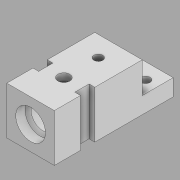
# Autodesk Inventor part: Box A01209499
Saved by Autodesk Inventor 2020 (Build 240168000, 168)
## iProperties
Created: 2019-10-15
Part Number: Box A01209499
Material: Genérico
Document SubType Name: Modeling
Designer: gerar
Density: 1 g/cm^3
Appearance: Valor por defecto
Author: gerar
Autodesk Inventor part; units mm, degrees
ref_plane "YZ Plane" through (0, 0, 0) normal (1, 0, 0) x (0, 1, 0)
ref_plane "XZ Plane" through (0, 0, 0) normal (0, 1, 0) x (-1, 0, 0)
ref_plane "XY Plane" through (0, 0, 0) normal (0, 0, 1) x (1, 0, 0)
sketch "Boceto1" plane through (0, 0, 0) normal (0, 1, 0) x (-1, 0, 0)
  line L0 (0, 0) -> (50.8, 0)
  line L1 (50.8, -93.98) -> (0, -93.98)
  line L2 (50.8, -27.94) -> (44.704, -27.94)
  line L3 (44.704, -27.94) -> (44.704, -43.18)
  line L4 (44.704, -43.18) -> (50.8, -43.18)
  line L5 (6.096, -27.94) -> (0, -27.94)
  line L6 (0, -43.18) -> (6.096, -43.18)
  line L7 (6.096, -43.18) -> (6.096, -27.94)
  line L8 (50.8, 0) -> (50.8, -27.94)
  line L9 (50.8, -43.18) -> (50.8, -93.98)
  line L10 (0, -93.98) -> (0, -43.18)
  line L11 (0, -27.94) -> (0, 0)
  dimension "d0" = 50.8
  dimension "d1" = 93.98
  dimension "d2" = 27.94
  dimension "d3" = 15.24
  dimension "d5" = 27.94
  dimension "d6" = 15.24
  constraints: 24 end point, 7 parallel, 3 horizontal, 3 perpendicular, 1 point on line
  measures "d0" distance of L1.start L1.end
  measures "d1" distance of L0.end L1.start
  measures "d2" distance between parallel lines of L0 L2
  measures "d3" distance between parallel lines of L2 L4
  measures "d5" distance between parallel lines of L0 L5
  measures "d6" distance between parallel lines of L6 L5
extrude "BaseAlta" add sketch "Boceto1" along normal blind 50.8
sketch "Boceto2" plane through (0, 0, 0) normal (0, 1, 0) x (-1, 0, 0)
  line L0 (0, -93.98) -> (50.8, -93.98) projected
  line L1 (0, -93.98) -> (50.8, -93.98)
  line L2 (50.8, -93.98) -> (50.8, -127)
  line L3 (50.8, -127) -> (0, -127)
  line L4 (0, -127) -> (0, -93.98)
  point P0 (0, 0)
  dimension "d10" = 50.8
  dimension "d11" = 33.02
  constraints: 8 end point, 2 parallel, 1 horizontal, 1 perpendicular
  measures "d10" distance of L2.end L3.end
  measures "d11" distance of L1.end L2.end
extrude "BaseBaja" add sketch "Boceto2" along normal blind 17.78
sketch "Boceto4" plane through (0, 50.8, -93.98) normal (0, 0, -1) x (-1, 0, 0)
  circle A0 centre (25.4, -25.4) radius 19.05 construction
  line L0 (0, -50.8) -> (50.8, -50.8) construction
  line L1 (0, -33.02) -> (0, 0) construction
  line L2 (6.35, -25.4) -> (15.875, -8.9022)
  line L3 (15.875, -8.9022) -> (34.925, -8.9022)
  line L4 (34.925, -8.9022) -> (44.45, -25.4)
  line L5 (44.45, -25.4) -> (34.925, -41.8978)
  line L6 (34.925, -41.8978) -> (15.875, -41.8978)
  line L7 (15.875, -41.8978) -> (6.35, -25.4)
  dimension "d19" = 38.1
  dimension "d20" = 25.4
  dimension "d21" = 25.4
  constraints: 12 end point, 1 coincident, 1 horizontal alignment, 15 other
  measures "d20" distance from line of L0 point (25.4, -25.4)
  measures "d21" distance from line of L1 point (25.4, -25.4)
extrude "Hexagono" cut sketch "Boceto4" against normal blind 43.18
sketch "Boceto6" plane through (0, 17.78, 0) normal (0, 1, 0) x (1, 0, 0)
  circle A0 centre (-38.1, 110.236) radius 4.826
  circle A1 centre (-12.7, 110.236) radius 4.826
  line L0 (0, 127) -> (-50.8, 127) projected
  line L1 (-50.8, 127) -> (-50.8, 93.98) projected
  line L2 (0, 93.98) -> (0, 127) projected
  point P0 (0, 0)
  dimension "d35" = 9.652
  dimension "d36" = 9.652
  dimension "d37" = 16.764
  dimension "d38" = 16.764
  dimension "d39" = 12.7
  dimension "d40" = 12.7
  dimension "d41" = 25.4
  constraints: 2 centre point
  measures "d35" diameter of A0
  measures "d36" diameter of A1
  measures "d37" distance from line of L0 A0.centre
  measures "d38" distance from line of L0 A1.centre
  measures "d39" distance from line of L1 A0.centre
  measures "d40" distance from line of L2 A1.centre
  measures "d41" distance of A1.centre A0.centre
extrude "DosAgujeros" cut sketch "Boceto6" against normal blind 10.16
sketch "Boceto7" plane through (0, 0, 0) normal (0, -1, 0) x (1, 0, 0)
  circle A0 centre (-12.7, -110.236) radius 4.826 construction
  circle A1 centre (-38.1, -110.236) radius 4.826 construction
  arc A2 (-12.7, -117.856) -> (-12.7, -102.616) centre (-12.7, -110.236) ccw
  arc A3 (-38.1, -102.616) -> (-38.1, -117.856) centre (-38.1, -110.236) ccw
  line L0 (-12.7, -117.856) -> (-38.1, -117.856)
  line L1 (-12.7, -102.616) -> (-38.1, -102.616)
  line L2 (0, -43.18) -> (0, -127) projected
  line L3 (0, -127) -> (-50.8, -127) projected
  line L4 (-50.8, -127) -> (-50.8, -43.18) projected
  point P0 (0, 0)
  dimension "d44" = 15.24
  dimension "d45" = 15.24
  dimension "d46" = 12.7
  dimension "d47" = 16.764
  dimension "d48" = 12.7
  dimension "d49" = 16.764
  constraints: 4 end point, 4 point on circle, 2 centre point, 2 coincident, 2 horizontal, 2 tangent
  measures "d44" diameter of A2
  measures "d45" diameter of A3
  measures "d46" distance from line of L2 A0.centre
  measures "d47" distance from line of L3 A0.centre
  measures "d48" distance from line of L4 A1.centre
  measures "d49" distance from line of L3 A1.centre
extrude "AgujeroInferior" cut sketch "Boceto7" against normal blind 7.62
sketch "Boceto8" plane through (-50.8, 0, 0) normal (0, 0, 1) x (1, 0, 0)
  line L0 (0, 0) -> (50.8, 0) projected
  line L1 (0, 0) -> (0, 50.8) projected
  point P0 (25.4, 25.4)
  dimension "d52" = 25.4
  dimension "d53" = 25.4
  measures "d52" distance from line of L0 point (25.4, 25.4)
  measures "d53" distance from line of L1 point (25.4, 25.4)
hole "Agujero" at (-25.4, 25.4, 0) direction (0, 0, -1) diameter 25.4 depth 50.8 tip angle 118 counterbore diameter 31.75 counterbore depth 13.208
sketch "Boceto9" plane through (0, 50.8, 0) normal (0, 1, 0) x (1, 0, 0)
  circle A0 centre (-25.4, 72.39) radius 4.7625
  line L0 (-50.8, 93.98) -> (-50.8, 43.18) projected
  line L1 (0, 93.98) -> (-50.8, 93.98) projected
  point P0 (0, 0)
  dimension "d61" = 9.525
  dimension "d62" = 25.4
  dimension "d63" = 21.59
  constraints: 1 centre point
  measures "d61" diameter of A0
  measures "d62" distance from line of L0 A0.centre
  measures "d63" distance from line of L1 A0.centre
extrude "HoyoSuperior" cut sketch "Boceto9" against normal blind 12.7
sketch "Boceto10" plane through (0, 50.8, 0) normal (0, 1, 0) x (1, 0, 0)
  line L0 (-50.8, 27.94) -> (-50.8, 0) projected
  line L1 (-50.8, 0) -> (0, 0) projected
  point P0 (-25.4, 35.56)
  dimension "d66" = 25.4
  dimension "d67" = 35.56
  measures "d66" distance from line of L0 point (-25.4, 35.56)
  measures "d67" distance from line of L1 point (-25.4, 35.56)
hole "Agujero3" at (-25.4, 50.8, -35.56) direction (0, -1, 0) diameter 7.874 depth 12.7 counterbore diameter 12.7 counterbore depth 7.62
chamfer "Chaflán1" distance 3.175 angle 45 1 edges at (-25.4, 41.275, -13.208) measured on face at (-24.1336, 10.7371, -13.208)
equation "\"d38\" = d37"
